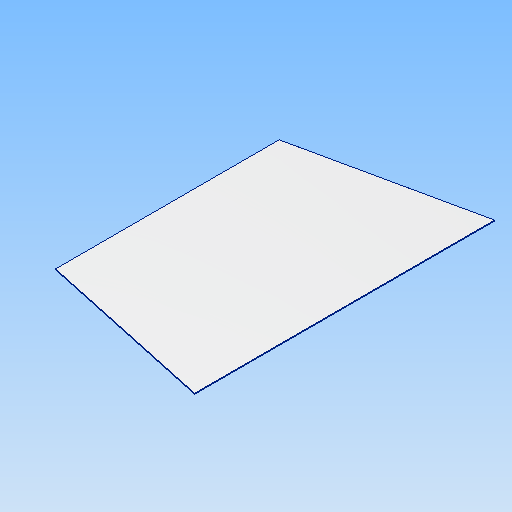
# Autodesk Inventor part: FirewallTrapezoid
Saved by Autodesk Inventor 2021 (Build 250183000, 183)
## iProperties
Created: 2020-10-17
Part Number: FirewallTrapezoid
Material: Aluminum 6061
Document SubType Name: Modeling
Designer: PhotonUser
Density: 2.7 g/cm^3
Appearance: Aluminum - Flat
Author: PhotonUser
Autodesk Inventor part; units mm, degrees
ref_plane "YZ Plane" through (0, 0, 0) normal (1, 0, 0) x (0, 1, 0)
ref_plane "XZ Plane" through (0, 0, 0) normal (0, 1, 0) x (-1, 0, 0)
ref_plane "XY Plane" through (0, 0, 0) normal (0, 0, 1) x (1, 0, 0)
sketch "Sketch2" plane through (0, 0, 0) normal (0, 1, 0) x (-1, 0, 0)
  line L0 (0, 0) -> (0, -558.8)
  line L1 (0, -558.8) -> (330.1969, -487.6803)
  line L2 (0, -558.8) -> (337.7692, -558.8) construction
  line L3 (330.1969, -487.6803) -> (330.1969, -71.1203)
  line L4 (330.1969, -71.1203) -> (0, 0)
  constraints: 10 end point, 2 vertical, 1 equal length, 1 horizontal
extrude "Extrusion1" add sketch "Sketch2" along normal blind 1.6002
body "Solid1"
